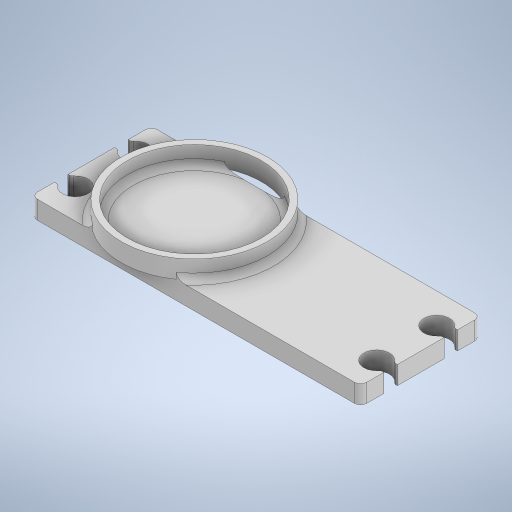
# Autodesk Inventor part: buh
Saved by Autodesk Inventor 2024 (Build 280153000, 153)
## iProperties
Created: 2024-02-05
Part Number: buh
Material: Generic
Document SubType Name: Modeling
Designer: jebes windows
Density: 1 g/cm^3
Appearance: Default
Author: jebes windows
Autodesk Inventor part; units mm, degrees
ref_plane "YZ Plane" through (0, 0, 0) normal (1, 0, 0) x (0, 1, 0)
ref_plane "XZ Plane" through (0, 0, 0) normal (0, 1, 0) x (-1, 0, 0)
ref_plane "XY Plane" through (0, 0, 0) normal (0, 0, 1) x (1, 0, 0)
sketch "Sketch1" plane through (0, 0, 0) normal (0, 0, 1) x (1, 0, 0)
  circle A0 centre (0, 0) radius 12
  line L0 (30.05, 0.475) -> (30.05, 9.55) projected
  line L1 (30.05, 0.475) -> (36.6, 0.475) projected
  line L2 (36.6, 0.475) -> (36.6, -0.475) projected
  line L3 (30.05, -0.475) -> (36.6, -0.475) projected
  line L4 (30.05, -9.55) -> (30.05, -0.475) projected
  arc A1 (29.75, -9.85) -> (30.05, -9.55) centre (29.75, -9.55) ccw projected
  line L5 (29.75, -9.85) -> (36.1, -9.85) projected
  arc A2 (36.1, -9.85) -> (37.1, -8.85) centre (36.1, -8.85) ccw projected
  line L6 (37.1, -8.85) -> (37.1, -6.025) projected
  line L7 (37.1, -6.025) -> (36.8605, -6.025) projected
  arc A3 (36.8605, -6.025) -> (36.4664, -6.2173) centre (36.8605, -6.525) ccw projected
  arc A4 (36.4664, -3.6327) -> (36.4664, -6.2173) centre (34.8111, -4.925) ccw projected
  arc A5 (36.4664, -3.6327) -> (36.8605, -3.825) centre (36.8605, -3.325) ccw projected
  line L8 (36.8605, -3.825) -> (37.1, -3.825) projected
  line L9 (37.1, -3.825) -> (37.1, 3.825) projected
  line L10 (37.1, 3.825) -> (36.8605, 3.825) projected
  arc A6 (36.8605, 3.825) -> (36.4664, 3.6327) centre (36.8605, 3.325) ccw projected
  arc A7 (36.4664, 6.2173) -> (36.4664, 3.6327) centre (34.8111, 4.925) ccw projected
  arc A8 (36.4664, 6.2173) -> (36.8605, 6.025) centre (36.8605, 6.525) ccw projected
  line L11 (36.8605, 6.025) -> (37.1, 6.025) projected
  line L12 (37.1, 6.025) -> (37.1, 8.85) projected
  arc A9 (37.1, 8.85) -> (36.1, 9.85) centre (36.1, 8.85) ccw projected
  line L13 (36.1, 9.85) -> (29.75, 9.85) projected
  arc A10 (30.05, 9.55) -> (29.75, 9.85) centre (29.75, 9.55) ccw projected
  line L14 (-16.4, 0.475) -> (-16.4, -0.475) projected
  line L15 (-9.85, 0.475) -> (-16.4, 0.475) projected
  line L16 (-9.85, 9.55) -> (-9.85, 0.475) projected
  arc A11 (-9.55, 9.85) -> (-9.85, 9.55) centre (-9.55, 9.55) ccw projected
  line L17 (-9.55, 9.85) -> (-15.9, 9.85) projected
  arc A12 (-15.9, 9.85) -> (-16.9, 8.85) centre (-15.9, 8.85) ccw projected
  line L18 (-16.9, 8.85) -> (-16.9, 6.025) projected
  line L19 (-16.9, 6.025) -> (-16.6605, 6.025) projected
  arc A13 (-16.6605, 6.025) -> (-16.2664, 6.2173) centre (-16.6605, 6.525) ccw projected
  arc A14 (-16.2664, 3.6327) -> (-16.2664, 6.2173) centre (-14.6111, 4.925) ccw projected
  arc A15 (-16.2664, 3.6327) -> (-16.6605, 3.825) centre (-16.6605, 3.325) ccw projected
  line L20 (-16.6605, 3.825) -> (-16.9, 3.825) projected
  line L21 (-16.9, 3.825) -> (-16.9, -3.825) projected
  line L22 (-16.9, -3.825) -> (-16.6605, -3.825) projected
  arc A16 (-16.6605, -3.825) -> (-16.2664, -3.6327) centre (-16.6605, -3.325) ccw projected
  arc A17 (-16.2664, -6.2173) -> (-16.2664, -3.6327) centre (-14.6111, -4.925) ccw projected
  arc A18 (-16.2664, -6.2173) -> (-16.6605, -6.025) centre (-16.6605, -6.525) ccw projected
  line L23 (-16.6605, -6.025) -> (-16.9, -6.025) projected
  line L24 (-16.9, -6.025) -> (-16.9, -8.85) projected
  arc A19 (-16.9, -8.85) -> (-15.9, -9.85) centre (-15.9, -8.85) ccw projected
  line L25 (-15.9, -9.85) -> (-9.55, -9.85) projected
  arc A20 (-9.85, -9.55) -> (-9.55, -9.85) centre (-9.55, -9.55) ccw projected
  line L26 (-9.85, -0.475) -> (-9.85, -9.55) projected
  line L27 (-9.85, -0.475) -> (-16.4, -0.475) projected
  line L28 (-9.55, 9.85) -> (29.75, 9.85)
  line L29 (29.75, -9.85) -> (-9.55, -9.85)
  circle A21 centre (0, 0) radius 11
  dimension "d0" = 24
  dimension "d1" = 1
  constraints: 4 end point, 2 centre point, 1 coincident, 1 collinear, 1 horizontal
  measures "d0" diameter of A0
  measures "d1" radial gap between concentric circles of A0 A21
extrude "Extrusion1" add sketch "Sketch1" along normal blind 3 contours A0 L29 A21 L28 | L28 A21 A0 | A0 L29 A21 | L28 A21 L16 A0 | A0 L26 A21 L29 | L16 A21 L15 A0 | A0 L27 A21 L26 | L15 A21 L27 A0
ref_plane "Work Plane1" through (0, 0, 0) normal (0, 0, 1) x (1, 0, 0)
sketch "Sketch2" plane through (0, 0, 0) normal (0, 0, 1) x (1, 0, 0)
  line L0 (-16.4, 0.475) -> (-16.4, -0.475) projected
  line L1 (-9.85, 0.475) -> (-16.4, 0.475) projected
  line L2 (-9.85, 9.55) -> (-9.85, 0.475) projected
  arc A0 (-9.55, 9.85) -> (-9.85, 9.55) centre (-9.55, 9.55) ccw projected
  line L3 (-9.55, 9.85) -> (-15.9, 9.85) projected
  arc A1 (-15.9, 9.85) -> (-16.9, 8.85) centre (-15.9, 8.85) ccw projected
  line L4 (-16.9, 8.85) -> (-16.9, 6.025) projected
  line L5 (-16.9, 6.025) -> (-16.6605, 6.025) projected
  arc A2 (-16.6605, 6.025) -> (-16.2664, 6.2173) centre (-16.6605, 6.525) ccw projected
  arc A3 (-16.2664, 3.6327) -> (-16.2664, 6.2173) centre (-14.6111, 4.925) ccw projected
  arc A4 (-16.2664, 3.6327) -> (-16.6605, 3.825) centre (-16.6605, 3.325) ccw projected
  line L6 (-16.6605, 3.825) -> (-16.9, 3.825) projected
  line L7 (-16.9, 3.825) -> (-16.9, -3.825) projected
  line L8 (-16.9, -3.825) -> (-16.6605, -3.825) projected
  arc A5 (-16.6605, -3.825) -> (-16.2664, -3.6327) centre (-16.6605, -3.325) ccw projected
  arc A6 (-16.2664, -6.2173) -> (-16.2664, -3.6327) centre (-14.6111, -4.925) ccw projected
  arc A7 (-16.2664, -6.2173) -> (-16.6605, -6.025) centre (-16.6605, -6.525) ccw projected
  line L9 (-16.6605, -6.025) -> (-16.9, -6.025) projected
  line L10 (-16.9, -6.025) -> (-16.9, -8.85) projected
  arc A8 (-16.9, -8.85) -> (-15.9, -9.85) centre (-15.9, -8.85) ccw projected
  line L11 (-15.9, -9.85) -> (-9.55, -9.85) projected
  arc A9 (-9.85, -9.55) -> (-9.55, -9.85) centre (-9.55, -9.55) ccw projected
  line L12 (-9.85, -0.475) -> (-9.85, -9.55) projected
  line L13 (-9.85, -0.475) -> (-16.4, -0.475) projected
  line L14 (30.05, 0.475) -> (30.05, 9.55) projected
  line L15 (30.05, 0.475) -> (36.6, 0.475) projected
  line L16 (36.6, 0.475) -> (36.6, -0.475) projected
  line L17 (30.05, -0.475) -> (36.6, -0.475) projected
  line L18 (30.05, -9.55) -> (30.05, -0.475) projected
  arc A10 (29.75, -9.85) -> (30.05, -9.55) centre (29.75, -9.55) ccw projected
  line L19 (29.75, -9.85) -> (36.1, -9.85) projected
  arc A11 (36.1, -9.85) -> (37.1, -8.85) centre (36.1, -8.85) ccw projected
  line L20 (37.1, -8.85) -> (37.1, -6.025) projected
  line L21 (37.1, -6.025) -> (36.8605, -6.025) projected
  arc A12 (36.8605, -6.025) -> (36.4664, -6.2173) centre (36.8605, -6.525) ccw projected
  arc A13 (36.4664, -3.6327) -> (36.4664, -6.2173) centre (34.8111, -4.925) ccw projected
  arc A14 (36.4664, -3.6327) -> (36.8605, -3.825) centre (36.8605, -3.325) ccw projected
  line L22 (36.8605, -3.825) -> (37.1, -3.825) projected
  line L23 (37.1, -3.825) -> (37.1, 3.825) projected
  line L24 (37.1, 3.825) -> (36.8605, 3.825) projected
  arc A15 (36.8605, 3.825) -> (36.4664, 3.6327) centre (36.8605, 3.325) ccw projected
  arc A16 (36.4664, 6.2173) -> (36.4664, 3.6327) centre (34.8111, 4.925) ccw projected
  arc A17 (36.4664, 6.2173) -> (36.8605, 6.025) centre (36.8605, 6.525) ccw projected
  line L25 (36.8605, 6.025) -> (37.1, 6.025) projected
  line L26 (37.1, 6.025) -> (37.1, 8.85) projected
  arc A18 (37.1, 8.85) -> (36.1, 9.85) centre (36.1, 8.85) ccw projected
  line L27 (36.1, 9.85) -> (29.75, 9.85) projected
  arc A19 (30.05, 9.55) -> (29.75, 9.85) centre (29.75, 9.55) ccw projected
  line L28 (29.75, 9.85) -> (-9.55, 9.85)
  line L29 (-9.55, -9.85) -> (29.75, -9.85)
  point P0 (0, 0)
  constraints: 4 end point, 2 horizontal
extrude "Extrusion2" add sketch "Sketch2" against normal blind 3
fillet "Fillet1" radius 1 3 edges at (10.636, 5.5566, 0) (10.636, -5.5566, 0) (-12, 0, 0)
fillet "Fillet2" radius 1 3 edges at (-11, 0, 0) (9.3505, 5.7938, 0) (9.3505, -5.7938, 0)
body "Solid1"
